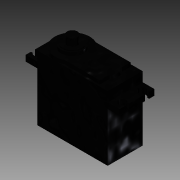
# Autodesk Inventor part: MG996RServo
Saved by Autodesk Inventor 2014 SP1 (Build 180222100, 222)
## iProperties
Created: 2017-01-17
Part Number: MG996RServo
Material: Generic
Document SubType Name: Modeling
Designer: danielsikar
Density: 1 g/cm^3
Appearance: Black
Author: danielsikar
Autodesk Inventor part; units mm, degrees
sketch "Sketch1" plane through (0, 0, 0) normal (0, 0, 1) x (1, 0, 0)
  line L0 (0, 0) -> (40.3, 0)
  line L1 (40.3, 0) -> (40.3, 20)
  line L2 (40.3, 20) -> (0, 20)
  line L3 (0, 20) -> (0, 0)
  dimension "d0" = 40.3
  dimension "d1" = 20
  constraints: 8 end point, 2 parallel, 1 horizontal, 1 perpendicular
  measures "d0" distance of L2.end L1.end
  measures "d1" distance of L1.end L0.end
extrude "Extrusion1" add sketch "Sketch1" along normal blind 37
sketch "Sketch2" plane through (40.3, 0, 0) normal (1, 0, 0) x (0, 0, -1)
  line L0 (0, 20) -> (-37, 20) projected
  line L1 (-37, 0) -> (-37, 20) projected
  line L2 (0, 0) -> (-37, 0) projected
  line L3 (-31.5, 0) -> (-28.2, 0)
  line L4 (-28.2, 0) -> (-28.2, 20)
  line L5 (-28.2, 20) -> (-31.5, 20)
  line L6 (-31.5, 20) -> (-31.5, 0)
  dimension "d4" = 3.3
  dimension "d5" = 5.5
  constraints: 8 end point, 2 parallel, 2 point on line, 1 horizontal, 1 perpendicular
  measures "d4" distance of L5.end L4.end
  measures "d5" distance between parallel lines of L6 L1
extrude "Extrusion2" add sketch "Sketch2" along normal blind 6.8 contours L4 L2 L6 L0
sketch "Sketch3" plane through (40.3, 0, 31.5) normal (0, 0, 1) x (1, 0, 0)
  line L0 (6.8, 20) -> (6.8, 0) projected
  line L1 (0, 20) -> (6.8, 20) projected
  circle A0 centre (4, 15.7) radius 2.2
  point P0 (-40.3, 0)
  dimension "d8" = 4.4
  dimension "d9" = 2.8
  dimension "d10" = 4.3
  constraints: 1 centre point
  measures "d8" diameter of A0
  measures "d9" distance from line of L0 A0.centre
  measures "d10" distance from line of A0.centre L1
extrude "Extrusion3" cut sketch "Sketch3" against normal through all
ref_plane "Work Plane2" through (48.1, 0, 0) normal (1, 0, 0) x (0, 0, -1)
sketch "Sketch7" plane through (48.1, 0, 0) normal (1, 0, 0) x (0, 0, -1)
  line L0 (-31.5, 16.9) -> (-28.2, 16.9) projected
  line L1 (-28.2, 14.5) -> (-31.5, 14.5) projected
  line L2 (-31.5, 16.9) -> (-28.2, 16.9)
  line L3 (-28.2, 16.9) -> (-28.2, 14.5)
  line L4 (-28.2, 14.5) -> (-31.5, 14.5)
  line L5 (-31.5, 14.5) -> (-31.5, 16.9)
  point P0 (0, 0)
  constraints: 8 end point, 2 parallel, 1 horizontal, 1 perpendicular
extrude "Extrusion5" cut sketch "Sketch7" against normal blind 3
ref_plane "Work Plane3" through (0, 10, 0) normal (0, 1, 0) x (-1, 0, 0)
mirror "Mirror1" about plane through (0, 10, 0) normal (0, 1, 0) of "Extrusion3", "Extrusion5"
ref_plane "Work Plane4" through (20.15, 0, 0) normal (1, 0, 0) x (0, 1, 0)
mirror "Mirror2" about plane through (20.15, 0, 0) normal (1, 0, 0) of "Extrusion2", "Extrusion3", "Extrusion5", "Mirror1"
sketch "Sketch8" plane through (0, 0, 37) normal (0, 0, 1) x (1, 0, 0)
  line L0 (40.3, 0) -> (40.3, 20) projected
  line L1 (40.3, 20) -> (0, 20) projected
  line L2 (0, 20) -> (0, 0) projected
  line L3 (34.6, 18.9) -> (14.5596, 18.9)
  line L4 (14.5596, 1.1) -> (34.6, 1.1)
  arc A0 (14.5596, 18.9) -> (14.5596, 1.1) centre (10, 10) ccw
  arc A1 (34.6, 6.0336) -> (34.6, 13.9664) centre (30.3, 10) ccw
  line L5 (34.6, 1.1) -> (34.6, 6.0336)
  line L6 (34.6, 13.9664) -> (34.6, 18.9)
  dimension "d27" = 1.1
  dimension "d29" = 20
  dimension "d30" = 10
  dimension "d31" = 11.7
  dimension "d32" = 10
  constraints: 8 end point, 4 point on circle, 2 centre point, 1 horizontal, 1 parallel
  measures "d27" distance between parallel lines of L3 L1
  measures "d29" diameter of A0
  measures "d30" distance from line of L2 A0.centre
  measures "d31" diameter of A1
  measures "d32" distance from line of L0 A1.centre
extrude "Extrusion6" add sketch "Sketch8" along normal blind 2 contours A0 L3 L6 A1 L5 L4
sketch "Sketch9" plane through (0, 0, 39) normal (0, 0, 1) x (1, 0, 0)
  arc A0 (14.5596, 18.9) -> (14.5596, 1.1) centre (10, 10) ccw projected
  circle A1 centre (10, 10) radius 6.5
  point P0 (0, 0)
  dimension "d35" = 13
  constraints: 1 centre point, 1 coincident
  measures "d35" diameter of A1
extrude "Extrusion7" add sketch "Sketch9" along normal blind 1.7
sketch "Sketch10" plane through (10, 10, 40.7) normal (0, 0, 1) x (1, 0, 0)
  circle A0 centre (0, 0) radius 6.5 projected
  circle A1 centre (0, 0) radius 5.55
  point P0 (-10, -10)
  dimension "d38" = 11.1
  constraints: 1 centre point, 1 coincident
  measures "d38" diameter of A1
extrude "Extrusion8" add sketch "Sketch10" along normal blind 0.4 contours A1
sketch "Sketch11" plane through (10, 10, 41.1) normal (0, 0, 1) x (1, 0, 0)
  circle A0 centre (0, 0) radius 5.55 projected
  circle A1 centre (0, 0) radius 2.95
  point P0 (-10, -10)
  dimension "d41" = 5.9
  constraints: 1 centre point, 1 coincident
  measures "d41" diameter of A1
extrude "Extrusion9" add sketch "Sketch11" along normal blind 4 contours A1
ref_plane "ConstraintPlane" through (10, 0, 0) normal (1, 0, 0) x (0, 1, 0)
body "Solid1"
